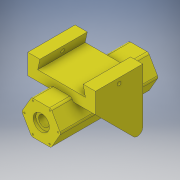
# Autodesk Inventor part: Nathan_Practice_5
Saved by Autodesk Inventor 2016 (Build 200138000, 138)
## iProperties
Created: 2017-03-08
Part Number: Nathan_Practice_5
Material: Generic
Document SubType Name: Modeling
Designer: Student
Density: 1 g/cm^3
Appearance: Default
Author: Student
Autodesk Inventor part; units mm, degrees
ref_plane "YZ Plane" through (0, 0, 0) normal (1, 0, 0) x (0, 1, 0)
ref_plane "XZ Plane" through (0, 0, 0) normal (0, 1, 0) x (-1, 0, 0)
ref_plane "XY Plane" through (0, 0, 0) normal (0, 0, 1) x (1, 0, 0)
sketch "Sketch1" plane through (0, 0, 0) normal (0, 0, 1) x (1, 0, 0)
  line L0 (7.2169, 12.5) -> (14.4338, 0)
  line L1 (14.4338, 0) -> (7.2169, -12.5)
  line L2 (7.2169, -12.5) -> (-7.2169, -12.5)
  line L3 (-7.2169, -12.5) -> (-14.4338, 0)
  line L4 (-14.4338, 0) -> (-7.2169, 12.5)
  line L5 (-7.2169, 12.5) -> (7.2169, 12.5)
  circle A0 centre (0, 0) radius 4
  dimension "d2" = 8
  dimension "d29" = 25
  constraints: 12 end point, 2 coincident, 1 centre point, 13 other
  measures "d2" diameter of A0
  measures "d29" distance between parallel lines of L2 L5
extrude "Extrusion1" add sketch "Sketch1" along normal blind 72
sketch "Sketch2" plane through (0, 0, 72) normal (0, 0, 1) x (1, 0, 0)
  circle A0 centre (0, 0) radius 6
  dimension "d5" = 12
  constraints: 1 centre point, 1 coincident
  measures "d5" diameter of A0
extrude "Extrusion2" cut sketch "Sketch2" against normal blind 2
sketch "Sketch3" plane through (0, 0, 72) normal (0, 0, 1) x (1, 0, 0)
  circle A0 centre (-12.4338, 0) radius 0.5175
  circle A1 centre (12.4338, 0) radius 0.5175
  line L0 (-7.2169, 12.5) -> (-14.4338, 0) projected
  line L1 (-14.4338, 0) -> (-7.2169, -12.5) projected
  line L2 (-7.2169, -12.5) -> (7.2169, -12.5) projected
  line L3 (7.2169, -12.5) -> (14.4338, 0) projected
  line L4 (14.4338, 0) -> (7.2169, 12.5) projected
  line L5 (7.2169, 12.5) -> (-7.2169, 12.5) projected
  circle A2 centre (0, 0) radius 4 projected
  line L6 (7.2169, -12.5) -> (-7.2169, -12.5) projected
  circle A3 centre (6.2412, 10.81) radius 0.5175
  circle A4 centre (-6.2526, 10.8298) radius 0.5175
  circle A5 centre (-6.2169, -10.6837) radius 0.5175
  circle A6 centre (6.1926, -10.7258) radius 0.5175
  dimension "d8" = 1.035
  dimension "d11" = 1.035
  dimension "d14" = 2
  dimension "d15" = 2
  dimension "d30" = 1.035
  dimension "d31" = 1.035
  dimension "d32" = 1.035
  dimension "d33" = 1.035
  constraints: 6 centre point
  measures "d8" diameter of A0
  measures "d11" diameter of A1
  measures "d14" distance of A0.centre L0.end
  measures "d15" distance of L3.end A1.centre
  measures "d30" diameter of A3
  measures "d31" diameter of A4
  measures "d32" diameter of A5
  measures "d33" diameter of A6
extrude "Extrusion3" cut sketch "Sketch3" against normal blind 4 contours A0 | A1 | A3 | A4 | A5 | A6
sketch "Sketch4" plane through (0, 0, 0) normal (1, 0, 0) x (0, 1, 0)
  line L0 (25, 57) -> (10, 57)
  line L1 (10, 22) -> (25, 22)
  line L2 (25, 22) -> (25, 57)
  line L3 (10, 22) -> (-25, 22)
  line L4 (-25, 22) -> (10, 57)
  line L5 (25, 22) -> (0, 22)
  line L6 (12.5, 0) -> (0, 0) projected
  line L7 (0, 0) -> (32, 0) construction
  line L8 (0, 0) -> (0, 72) projected
  dimension "d20" = 15
  dimension "d21" = 35
  dimension "d22" = 35
  dimension "d27" = 25
  dimension "d47" = 22
  dimension "d48" = 25
  dimension "d49" = 45
  constraints: 14 end point, 2 horizontal, 1 collinear, 1 parallel, 1 point on line
  measures "d20" distance of L1.end L1.start
  measures "d21" distance of L1.start L0.end
  measures "d22" distance of L1.start L3.end
  measures "d27" distance of L1.end L5.end
  measures "d47" distance between parallel lines of L7 L1
  measures "d48" distance between parallel lines of L2 L8
  measures "d49" angle of L3 L4
extrude "Extrusion4" add sketch "Sketch4" along normal mid plane 50
fillet "Fillet1" radius 4 1 edges at (0, -25, 22)
fillet "Fillet2" radius 2 12 edges at (-7.2169, -12.5, 53.25) (7.2169, -12.5, 53.25) (14.4338, 0, 59.5) (-14.4338, 0, 59.5) (-7.2169, 12.5, 64.5) (7.2169, 12.5, 64.5) (-14.4338, 0, 11) (-7.2169, 12.5, 11) (-7.2169, -12.5, 11) (7.2169, 12.5, 11) (14.4338, 0, 11) (7.2169, -12.5, 11)
sketch "Sketch5" plane through (-25, 25, 57) normal (0, 0, 1) x (1, 0, 0)
  line L0 (0, -15) -> (0, 0) projected
  line L1 (0, 0) -> (9, 0)
  line L2 (50, 0) -> (0, 0) projected
  line L3 (50, 0) -> (50, -15) projected
  line L4 (50, 0) -> (41, 0)
  line L5 (41, 0) -> (42.5942, -7.5)
  line L6 (41, 0) -> (48.6676, 0) construction
  line L7 (9, 0) -> (7.4058, -7.5)
  line L8 (9, 0) -> (16.6676, 0) construction
  line L9 (7.4058, -7.5) -> (42.5942, -7.5)
  line L10 (9, 0) -> (41, 0)
  point P0 (25, -25)
  dimension "d35" = 9
  dimension "d37" = 78
  dimension "d38" = 102
  constraints: 16 end point, 3 horizontal, 2 equal length, 2 point on line, 1 collinear
  measures "d35" distance of L2.start L4.end
  measures "d37" angle of L5 L6
  measures "d38" angle of L7 L8
extrude "Extrusion5" cut sketch "Sketch5" along normal mid plane 500
sketch "Sketch6" plane through (-25, 0, 0) normal (-1, 0, 0) x (0, 0, 1)
  line L0 (57, 25) -> (22, 25) projected
  line L1 (22, 25) -> (39.5, 25)
  line L2 (39.5, 25) -> (39.5, 17.5)
  line L3 (22, 17.5) -> (57, 17.5) projected
  circle A0 centre (39.5, 21.25) radius 1.4
  point P0 (0, 0)
  dimension "d41" = 17.5
  dimension "d42" = 2.8
  constraints: 4 end point, 3 midpoint, 1 centre point
  measures "d41" distance of L0.end L1.end
  measures "d42" diameter of A0
extrude "Extrusion6" cut sketch "Sketch6" against normal blind 70
sketch "Sketch8" plane through (0, 0, 72) normal (0, 0, 1) x (1, 0, 0)
  circle A0 centre (0, 0) radius 4 projected
  circle A1 centre (0, 0) radius 4
  constraints: 1 centre point, 1 coincident
extrude "Extrusion8" cut sketch "Sketch8" against normal blind 70
body "Solid1"
